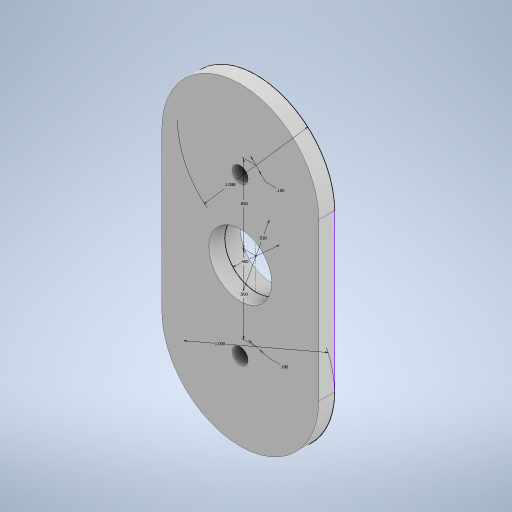
# Autodesk Inventor part: bearing_bracket_cover
Saved by Autodesk Inventor 2024 (Build 280153000, 153)
## iProperties
Created: 2023-11-30
Part Number: bearing_bracket_cover
Material: Generic
Document SubType Name: Modeling
Designer: jerem
Density: 1 g/cm^3
Appearance: Default
Author: jerem
## iProperties of the stored document bearing_bracket_cover_3DPrint.ipt
Created: 2023-11-30
Part Number: bearing_bracket_cover_3DPrint
Material: Generic
Document SubType Name: Modeling
Designer: jerem
Density: 1 g/cm^3
Appearance: Default
Author: jerem
Autodesk Inventor part; units mm, degrees
ref_plane "YZ Plane" through (0, 0, 0) normal (1, 0, 0) x (0, 1, 0)
ref_plane "XZ Plane" through (0, 0, 0) normal (0, 1, 0) x (-1, 0, 0)
ref_plane "XY Plane" through (0, 0, 0) normal (0, 0, 1) x (1, 0, 0)
sketch "Sketch1" plane through (0, 0, 0) normal (0, 0, 1) x (1, 0, 0)
  line L0 (0, 0) -> (0, 12.7) construction
  line L1 (0, 0) -> (0, -12.7) construction
  circle A0 centre (0, 12.7) radius 1.27
  circle A1 centre (0, -12.7) radius 1.27
  arc A2 (12.7, 12.7) -> (-12.7, 12.7) centre (0, 12.7) ccw
  arc A3 (-12.7, -12.7) -> (12.7, -12.7) centre (0, -12.7) ccw
  line L2 (-12.7, -12.7) -> (-12.7, 12.7)
  line L3 (12.7, 12.7) -> (12.7, -12.7)
  circle A4 centre (0, 0) radius 6.477
  circle A5 centre (0, 0) radius 5.08
  dimension "d0" = 12.7
  dimension "d1" = 12.7
  dimension "d2" = 2.54
  dimension "d3" = 2.54
  dimension "d4" = 25.4
  dimension "d5" = 25.4
  dimension "d6" = 12.954
  dimension "d7" = 10.16
  constraints: 8 end point, 6 centre point, 6 coincident, 4 point on circle, 3 vertical, 2 tangent
  measures "d0" distance of L0.start L0.end
  measures "d1" distance of L0.start L1.end
  measures "d2" diameter of A0
  measures "d3" diameter of A1
  measures "d4" diameter of A2
  measures "d5" diameter of A3
  measures "d6" diameter of A4
  measures "d7" diameter of A5
extrude "Extrusion1" add sketch "Sketch1" along normal blind 2.54 contours L3 A3 L2 A2 | A4
extrude "Extrusion2" add sketch "Sketch1" against normal blind 2.54 contours A4
body "Solid1"
